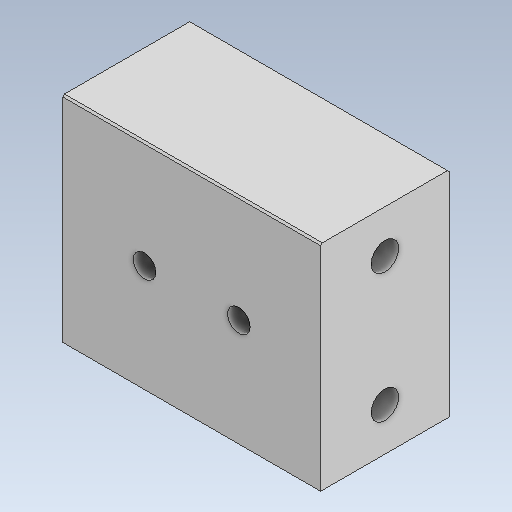
# Autodesk Inventor part: Soporte mesa
Saved by Autodesk Inventor 2021 (Build 250183000, 183)
## iProperties
Created: 2021-05-29
Part Number: Soporte mesa
Material: Generic
Document SubType Name: Modeling
Designer: Nelson
Density: 1 g/cm^3
Appearance: Default
Author: Nelson
Autodesk Inventor part; units mm, degrees
ref_plane "YZ Plane" through (0, 0, 0) normal (1, 0, 0) x (0, 1, 0)
ref_plane "XZ Plane" through (0, 0, 0) normal (0, 1, 0) x (-1, 0, 0)
ref_plane "XY Plane" through (0, 0, 0) normal (0, 0, 1) x (1, 0, 0)
sketch "Sketch1" plane through (0, 0, 0) normal (0, 0, 1) x (1, 0, 0)
  line L0 (0, 0) -> (300.8, 0)
  line L1 (300.8, 0) -> (300.8, 250)
  line L2 (300.8, 250) -> (0, 250)
  line L3 (0, 250) -> (0, 0)
  dimension "d0" = 300.8
  dimension "d1" = 250
  constraints: 8 end point, 2 parallel, 1 horizontal, 1 perpendicular
  measures "d0" distance of L1.end L2.end
  measures "d1" distance of L0.end L1.end
extrude "Extrusion1" add sketch "Sketch1" against normal blind 150
sketch "Sketch2" plane through (300.8, 0, 0) normal (1, 0, 0) x (0, 0, -1)
  line L0 (0, 0) -> (0, 250) projected
  line L1 (0, 250) -> (150, 250) projected
  point P0 (75, 200)
  point P1 (75, 50)
  dimension "d4" = 75
  dimension "d5" = 75
  dimension "d6" = 150
  dimension "d7" = 50
  measures "d4" distance from line of point (75, 200) L0
  measures "d5" distance from line of point (75, 50) L0
  measures "d6" distance of point (75, 50) point (75, 200)
  measures "d7" distance from line of L1 point (75, 200)
hole "Hole1" at (300.8, 200, -75) at (300.8, 50, -75) direction (-1, 0, 0) diameter 32 end through all
sketch "Sketch3" plane through (0, 0, 0) normal (0, 0, 1) x (1, 0, 0)
  line L0 (0, 0) -> (300.8, 0) projected
  line L1 (300.8, 250) -> (0, 250) projected
  line L2 (0, 250) -> (0, 0) projected
  line L3 (300.8, 0) -> (300.8, 250) projected
  point P0 (95.4, 125)
  point P1 (205.4, 125)
  dimension "d16" = 125
  dimension "d17" = 125
  dimension "d31" = 110
  dimension "d32" = 95.4
  measures "d16" distance from line of point (95.4, 125) L1
  measures "d17" distance from line of L1 point (205.4, 125)
  measures "d31" distance of point (205.4, 125) point (95.4, 125)
  measures "d32" distance from line of point (95.4, 125) L2
hole "Hole2" at (95.4, 125, 0) at (205.4, 125, 0) direction (0, 0, -1) diameter 26.4 end through all
chamfer "Chamfer1" distance 2 angle 45 2 edges at (150.4, 250, -150) (150.4, 250, 0)
equation "\"d5\" = d4"
equation "\"d17\" = d16"
body "Solid1"
